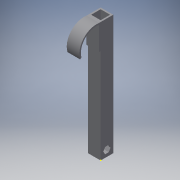
# Autodesk Inventor part: claw
Saved by Autodesk Inventor 2016 (Build 200138000, 138)
## iProperties
Created: 2016-02-22
Part Number: claw
Material: Generic
Document SubType Name: Modeling
Designer: Admin
Density: 1 g/cm^3
Appearance: Default
Author: Admin
Autodesk Inventor part; units mm, degrees
ref_plane "YZ Plane" through (0, 0, 0) normal (1, 0, 0) x (0, 1, 0)
ref_plane "XZ Plane" through (0, 0, 0) normal (0, 1, 0) x (-1, 0, 0)
ref_plane "XY Plane" through (0, 0, 0) normal (0, 0, 1) x (1, 0, 0)
sketch "Sketch1" plane through (0, 0, 0) normal (1, 0, 0) x (0, 1, 0)
  line L0 (0, 0) -> (241.3, 0)
  line L1 (241.3, 0) -> (241.3, -25.4)
  line L2 (241.3, -25.4) -> (0, -25.4)
  line L3 (0, -25.4) -> (0, 0)
  line L4 (6.3489, -9.0357) -> (12.6978, -5.3677)
  line L5 (12.6978, -5.3677) -> (19.0489, -9.0319)
  line L6 (19.0489, -9.0319) -> (19.0511, -16.3643)
  line L7 (19.0511, -16.3643) -> (12.7022, -20.0323)
  line L8 (12.7022, -20.0323) -> (6.3511, -16.3681)
  line L9 (6.3511, -16.3681) -> (6.3489, -9.0357)
  point P0 (12.7, -12.7)
  dimension "d0" = 241.3
  dimension "d1" = 25.4
  dimension "d3" = 12.7
  dimension "d4" = 12.7
  constraints: 20 end point, 2 parallel, 1 horizontal, 1 perpendicular, 13 other
  measures "d0" distance of L1.end L2.end
  measures "d1" distance of L0.end L1.end
  measures "d3" distance between parallel lines of L9 L6
  measures "d4" distance from line of L3 point (12.7, -12.7)
extrude "Extrusion1" add sketch "Sketch1" along normal blind 25.4
sketch "Sketch2" plane through (0, 241.3, 0) normal (0, 1, 0) x (1, 0, 0)
  line L0 (0, 25.4) -> (25.4, 25.4) projected
  line L1 (0, 0) -> (25.4, 0)
  line L2 (25.4, 0) -> (25.4, 25.4)
  line L3 (25.4, 25.4) -> (0, 25.4)
  line L4 (0, 25.4) -> (0, 0)
  line L5 (22.225, 3.175) -> (3.175, 3.175)
  line L6 (3.175, 3.175) -> (3.175, 22.225)
  line L7 (3.175, 22.225) -> (22.225, 22.225)
  line L8 (22.225, 22.225) -> (22.225, 3.175)
  dimension "d7" = 3.175
  constraints: 16 end point, 4 parallel, 2 perpendicular, 1 horizontal, 3 other
  measures "d7" distance between parallel lines of L1 L5
extrude "Extrusion2" cut sketch "Sketch2" against normal blind 228.6 contours L5 L6 L7 L8
sketch "Sketch3" plane through (25.4, 0, 0) normal (1, 0, 0) x (0, 0, -1)
  line L0 (0, 241.3) -> (0, 190.5)
  line L1 (0, 0) -> (0, 241.3) projected
  line L2 (0, 241.3) -> (-3.175, 241.3)
  line L3 (-3.175, 241.3) -> (-3.175, 190.5)
  line L4 (-3.175, 190.5) -> (0, 190.5)
  line L5 (0, 190.5) -> (0, 241.3)
  arc A0 (-3.175, 241.3) -> (-46.143, 196.9282) centre (-8.4506, 203.4185) ccw
  line L6 (-3.175, 241.3) -> (-3.175, 238.125)
  arc A1 (-3.175, 238.125) -> (-42.9327, 197.9157) centre (-7.6224, 202.7623) ccw
  line L7 (-42.9327, 197.9157) -> (-46.143, 196.9282)
  dimension "d11" = 50.8
  dimension "d13" = 3.175
  dimension "d15" = 3.175
  constraints: 14 end point, 4 point on circle, 2 centre point, 2 parallel, 2 point on line, 1 horizontal, 1 perpendicular
  measures "d11" distance of L0.start L0.end
  measures "d13" distance of L4.end L3.end
  measures "d15" distance of L2.end L6.end
extrude "Extrusion3" add sketch "Sketch3" against normal blind 25.4 contours L0 L4 L3 L2
sketch "Sketch4" plane through (25.4, 0, 0) normal (1, 0, 0) x (0, 0, -1)
  point P0 (0, 0)
sketch "Sketch5" plane through (25.4, 0, 0) normal (1, 0, 0) x (0, 0, -1)
  line L0 (-3.175, 241.3) -> (-3.175, 190.5) projected
  line L1 (-3.175, 241.3) -> (-3.175, 196.85)
  line L2 (-3.175, 196.85) -> (-41.275, 196.85)
  arc A0 (-3.175, 241.3) -> (-41.275, 196.85) centre (-8.1247, 206.989) ccw
  line L3 (-41.275, 196.85) -> (-38.5091, 198.4089)
  line L4 (-3.175, 241.3) -> (-3.175, 238.125)
  arc A1 (-3.175, 238.125) -> (-38.5091, 198.4089) centre (-8.433, 207.227) ccw
  point P0 (0, 0)
  dimension "d18" = 44.45
  dimension "d19" = 38.1
  dimension "d20" = 3.175
  dimension "d21" = 3.175
  constraints: 8 end point, 4 point on circle, 2 centre point, 2 point on line, 1 perpendicular
  measures "d18" distance of L0.start L1.end
  measures "d19" distance of L1.end L2.end
  measures "d20" distance of L2.end L3.end
  measures "d21" distance of L0.start L4.end
extrude "Extrusion4" add sketch "Sketch5" against normal blind 25.4 contours L0 A1 L3 A0
sketch "Sketch6" plane through (25.4, 0, 0) normal (1, 0, 0) x (0, 0, -1)
  line L0 (0, 0) -> (25.4, 0) projected
  line L1 (25.4, 0) -> (25.4, 241.3) projected
  line L2 (12.7618, 20.0321) -> (19.0807, 16.3125)
  line L3 (19.0807, 16.3125) -> (19.0189, 8.9804)
  line L4 (19.0189, 8.9804) -> (12.6382, 5.3679)
  line L5 (12.6382, 5.3679) -> (6.3193, 9.0875)
  line L6 (6.3193, 9.0875) -> (6.3811, 16.4196)
  line L7 (6.3811, 16.4196) -> (12.7618, 20.0321)
  point P0 (12.7, 12.7)
  point P1 (12.7, 12.7)
  dimension "d25" = 12.7
  dimension "d26" = 12.7
  dimension "d27" = 12.7
  constraints: 12 end point, 1 coincident, 13 other
  measures "d25" distance from line of L0 point (12.7, 12.7)
  measures "d26" distance from line of L1 point (12.7, 12.7)
  measures "d27" distance between parallel lines of L5 L2
extrude "Extrusion5" cut sketch "Sketch6" against normal blind 25.4
body "Solid1"
